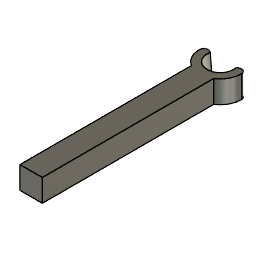
expoxy sticks_v4 (Autodesk Fusion 360 design; units mm, degrees)
Autodesk Fusion 360 part; units mm, degrees
sketch "Sketch1" plane through (0, 0, 0) normal (0, 0, 1) x (1, 0, 0)
  circle A0 centre (0, 0) radius 2.75
  circle A1 centre (0, 0) radius 7.5
  line L0 (0, 0) -> (7.5, 0) construction
  line L1 (0, 0) -> (-7.5, 0) construction
  line L2 (-2.75, 0) -> (-7.0726, 2.4957)
  line L3 (0, 0) -> (0, 7.5)
  line L4 (2.75, 0) -> (7.0726, 2.4957)
  line L5 (0, -7.5) -> (0, -67.5)
  line L6 (-5, -67.5) -> (5, -67.5)
  line L7 (5, -67.5) -> (7.4948, -0.2782)
  line L8 (-5, -67.5) -> (-7.4948, -0.2782)
  line L9 (15, 0) -> (22, 0)
  line L10 (22, 0) -> (22, -70)
  line L11 (22, -70) -> (15, -70)
  line L12 (15, -70) -> (15, 0)
  dimension "d1" = 5.5
  dimension "d2" = 15
  dimension "d3" = 150
  dimension "d4" = 60
  dimension "d11" = 7
  dimension "d12" = 70
  constraint coincident A0.centre A1.centre
  constraint concentric A0 A1
  constraint coincident A1 L0.end
  constraint horizontal L0
  constraint coincident A1 L1.end
  constraint parallel L0 L1
  constraint coincident L1 L2.start
  constraint coincident A0 L2.start
  constraint coincident A1 L2.end
  constraint coincident A1 L3.end
  constraint perpendicular L1 L3
  constraint symmetric L2.start L3 L4.start
  constraint symmetric L2.end L3 L4.end
  constraint coincident A1 L5.start
  constraint parallel L3 L5
  constraint midpoint L5.end L6
  constraint perpendicular L5 L6
  constraint coincident A1 L7.end
  constraint tangent A1 L7
  constraint coincident A1 L8.end
  constraint tangent A1 L8
  constraint horizontal L9
  constraint vertical L10
  constraint horizontal L11
  constraint vertical L12
  measures "d1" diameter of A0
  measures "d2" diameter of A1
  measures "d3" angle of L1 L2
  measures "d4" distance of L5.start L5.end
  measures "d11" distance of L9.start L9.end
  measures "d12" distance of L9.start L11.end
extrude "Extrude1" add sketch "Sketch1" along normal blind 8 contours A0 A1 L2 L4 | A1 L5 L6 L8 | A1 L5 L6 L7 | L9 L10 L11 L12 makes body 1 at (0.0685, -45.9141, 0) makes body 2 at (22, -23.3333, 5.3333)
fillet "Fillet1" radius 1.5 2 edges at (-7.0726, 2.4957, 4) (7.0726, 2.4957, 4) on bodies 1
chamfer "Chamfer1" distance 2 distance2 8 1 edges at (0, -2.75, 8) measured on face at (0.0685, -45.9141, 8) tangent chain off on bodies 1
chamfer "Chamfer2" distance 2 distance2 8 1 edges at (18.5, 0, 8) measured on face at (19.6667, -46.6667, 8) tangent chain off on bodies 2
sketch "Sketch2" plane through (0, 0, 0) normal (0, 0, -1) x (1, 0, 0)
  arc A0 (5.2483, -1.4424) -> (7.4979, -0.1792) centre (5.9983, -0.1433) ccw
  arc A1 (7.4979, -0.1792) -> (7.4948, 0.2782) centre (0, 0) ccw
  line L0 (7.4948, 0.2782) -> (5, 67.5)
  line L1 (5, 67.5) -> (-5, 67.5)
  line L2 (-5, 67.5) -> (-7.4948, 0.2782)
  arc A2 (-7.4948, 0.2782) -> (-7.4979, -0.1792) centre (0, 0) ccw
  arc A3 (-7.4979, -0.1792) -> (-5.2483, -1.4424) centre (-5.9983, -0.1433) ccw
  line L3 (-5.2483, -1.4424) -> (-2.75, 0)
  arc A4 (2.75, 0) -> (-2.75, 0) centre (0, 0) ccw
  line L4 (2.75, 0) -> (5.2483, -1.4424)
  circle A5 centre (0, 0) radius 7.5
  line L5 (0, 67.5) -> (-3.9972, 67.6484)
  line L6 (-3.9972, 67.6484) -> (-3.9972, 6.346)
  line L7 (0, 67.5) -> (4, 67.5)
  line L8 (4, 67.5) -> (4, 6.3443)
  dimension "d15" = 4
  dimension "d16" = 4
  constraint concentric A1 A5
  constraint coincident A1.end A5
  constraint midpoint L1 L5.start
  constraint perpendicular L2 L5
  constraint coincident A5 L6.end
  constraint vertical L6
  constraint coincident L1 L7.end
  constraint coincident A5 L8.end
  constraint perpendicular L7 L8
  measures "d15" distance of L5.start L5.end
  measures "d16" distance of L5.start L7.end
extrude "Extrude2" cut sketch "Sketch2" against normal blind 18 contours L0 L1 A5 L8 | L1 L2 A5 L6 bodies 1
hidden bodies 2
